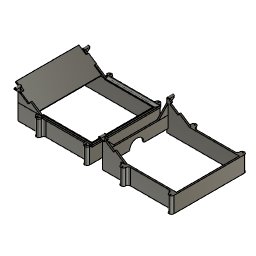
Led backlight edge holder (Autodesk Fusion 360 design; units mm, degrees)
Autodesk Fusion 360 part; units mm, degrees
note: some values were not read from the file. Chosen so that the rebuilt part matches the saved one: which pieces of a blend or face edit are solid. Set by a fixed rule: which sketch regions a step uses.
sketch "Sketch1" plane through (0, 0, 0) normal (0, 0, 1) x (1, 0, 0) in component "Base"
  line L0 (110, 0) -> (110, 126)
  line L1 (110, 126) -> (0, 126)
  line L2 (0, 126) -> (0, 0)
  line L3 (112, 128) -> (-35, 128)
  line L4 (-35, 128) -> (-35, -2)
  line L5 (-35, -2) -> (112, -2)
  line L6 (112, -2) -> (112, 128)
  line L7 (-45, 126) -> (-45, 0)
  line L8 (0, 0) -> (0, 126)
  line L9 (115, 131) -> (-38, 131)
  line L10 (-38, 131) -> (-38, -5)
  line L11 (-38, -5) -> (115, -5)
  line L12 (115, -5) -> (115, 131)
  line L13 (-35, -2) -> (-38, -2)
  line L14 (-35, 128) -> (-38, 128)
  line L15 (-38, 0) -> (-45, 0)
  line L16 (-45, 0) -> (-45, 126)
  line L17 (-45, 126) -> (-38, 126)
  line L18 (110, 0) -> (0, 0)
  line L19 (115, -5) -> (105, -5)
  line L20 (105, -5) -> (105, -15)
  line L21 (105, -15) -> (115, -15)
  line L22 (115, -15) -> (115, -5)
  line L23 (115, 131) -> (105, 131)
  line L24 (105, 131) -> (105, 141)
  line L25 (105, 141) -> (115, 141)
  line L26 (115, 141) -> (115, 131)
  line L27 (15, -5) -> (5, -5)
  line L28 (5, -5) -> (5, -15)
  line L29 (5, -15) -> (15, -15)
  line L30 (15, -15) -> (15, -5)
  line L31 (5, 131) -> (5, 141)
  line L32 (5, 141) -> (15, 141)
  line L33 (15, 141) -> (15, 131)
  line L34 (15, 131) -> (5, 131)
  circle A0 centre (10, -12) radius 1
  circle A1 centre (110, -12) radius 1
  circle A2 centre (110, 138) radius 1
  circle A3 centre (10, 138) radius 1
  dimension "d4" = 110
  dimension "d5" = 126
  dimension "d8" = 147
  dimension "d9" = 130
  dimension "d11" = 153
  dimension "d12" = 136
  constraint vertical L0
  constraint horizontal L1
  constraint vertical L2
  constraint coincident L2.end L8.start
  constraint horizontal L3
  constraint vertical L4
  constraint horizontal L5
  constraint vertical L6
  constraint vertical L7
  constraint vertical L8
  constraint horizontal L9
  constraint vertical L10
  constraint horizontal L11
  constraint vertical L12
  constraint coincident L10 L13.end
  constraint perpendicular L10 L13
  constraint coincident L10 L14.end
  constraint perpendicular L10 L14
  constraint coincident L10 L15.start
  constraint coincident L10 L17.end
  constraint perpendicular L2 L18
  constraint horizontal L19
  constraint vertical L20
  constraint horizontal L21
  constraint vertical L22
  constraint horizontal L23
  constraint vertical L24
  constraint horizontal L25
  constraint vertical L26
  constraint horizontal L27
  constraint vertical L28
  constraint horizontal L29
  constraint vertical L30
  constraint horizontal L34
  constraint vertical L31
  constraint horizontal L32
  constraint vertical L33
  measures "d4" distance of L2.end L0.start
  measures "d5" distance of L2.end L1.end
  measures "d8" distance of L3.start L3.end
  measures "d9" distance of L3.start L5.end
  measures "d11" distance of L9.start L9.end
  measures "d12" distance of L9.start L11.end
extrude "Extrude1" add sketch "Sketch1" along normal blind 30 contours L3 L5 L6 L9 L10 L11 L12 L13 L14 L19 L23 L27 L34 makes body 1 in component "Base"
extrude "Extrude2" add sketch "Sketch1" along normal blind 30 contours L4 L10 L13 L14 bodies 1 in component "Base"
extrude "Extrude3" cut sketch "Sketch1" along normal blind 6 contours L4 L10 L13 L14 bodies 1 in component "Base"
sketch "Sketch2" plane through (0, 131, 0) normal (0, 1, 0) x (-1, 0, 0) in component "Ramp holder"
  line L0 (-115, 0) -> (38, 0)
  line L1 (38, 0) -> (38, 30)
  line L2 (38, 30) -> (-115, 30)
  line L3 (-115, 30) -> (-115, 0)
  line L4 (14.7979, 39.9099) -> (31.5016, 50.9092)
  line L5 (14.7979, 39.9099) -> (12.048, 44.0859)
  line L6 (31.5016, 50.9092) -> (28.7518, 55.0852)
  circle A0 centre (35.72, 59.5131) radius 0.9615
  circle A1 centre (35.72, 59.5131) radius 1.3
  circle A2 centre (35.72, 59.5131) radius 2.3
  line L7 (38.02, 57.0131) -> (38.0199, 59.4994)
  line L8 (33.42, 57.0131) -> (33.42, 59.5131)
  line L9 (33.42, 57.0131) -> (38.02, 57.0131)
  line L10 (38, 30, 0) -> (38, 30, -136)
  line L11 (38, 30, 0) -> (38, 30, -23)
  line L12 (38, 30) -> (-9.3431, 30)
  line L13 (-9.3431, 30) -> (12.048, 44.0859)
  line L14 (38, 30) -> (38.0199, 30.0131)
  line L15 (38, 30) -> (38.02, 57.0131)
  line L16 (28.7518, 55.0852) -> (33.42, 58.1591)
  line L17 (38.0155, 50.9044, 0) -> (38.0155, 50.9044, -3)
  line L18 (38.0155, 50.9044, -3) -> (38, 30, -23)
  line L19 (38, 30) -> (38.0155, 50.9044)
  dimension "d28" = 5
  dimension "d67" = 23
  dimension "d98" = 3
  constraint concentric A0 A1
  constraint concentric A1 A2
  constraint coincident A2 L7.end
  constraint coincident A2 L8.end
  constraint tangent A2 L8
  constraint horizontal L9
  constraint coincident L1.end L2.start
  constraint coincident L2 L12.end
  constraint perpendicular L5 L13
  constraint coincident L8 L16.end
  constraint coincident L15 L19.end
  measures "d28" distance of L4.end L6.end
  measures "d67" distance of L1.end L2.start
extrude "Extrude5" add sketch "Sketch2" against normal blind 3 separate body contours L2 L4 L5 L6 L8 L9 L12 L13 L15 L16 L19 | A2 L7 L8 L9 | A2 | A1 makes body 2 in component "Base"
extrude "Extrude6" cut sketch "Sketch2" against normal blind 2 contours A1 bodies 2 in component "Base"
extrude "Extrude7" add sketch "Sketch2" along normal blind 8 contours A2 L7 L8 L9 | A2 bodies 2 in component "Base"
fillet "Fillet3" radius 8 tangency weight 0.3 1 edges at (-35.72, 131, 57.0131) on bodies 2 in component "Base"
fillet "Fillet2" radius 1.25 tangency weight 0.8 1 edges at (-35.72, 139, 57.0131) on bodies 2 in component "Base"
sketch "Sketch2 (curves on the plane with normal -1, 0, -0.0007 at 37.9778 mm)" plane through (-37.9778, 131, -0.0281) normal (-1, 0, -0.00074) x (-0.00074, 0, 1)
  line L0 (30.0281, 0) -> (30.0281, -136)
  line L1 (30.0281, 0) -> (30.0281, -23)
  line L2 (30.0281, 0) -> (57.0412, 0)
  line L3 (50.9325, 0) -> (50.9325, -3)
  line L4 (50.9325, -3) -> (30.0281, -23)
  line L5 (30.0281, 0) -> (50.9325, 0)
extrude "Extrude9" add sketch "Sketch2 (curves on the plane with normal -1, 0, -0.0007 at 37.9778 mm)" against normal blind 3 bodies 2 in component "Base"
sketch "Sketch1 (2)" plane through (0, 0, 0) normal (0, 0, 1) x (1, 0, 0) in component "Ramp"
  line L0 (-78, 135) -> (-78, 140)
  line L1 (-78, 140) -> (-98, 140)
  line L2 (-98, 140) -> (-98, 135)
  line L3 (-98, 5) -> (-98, 0)
  line L4 (-98, 0) -> (-78, 0)
  line L5 (-78, 0) -> (-78, 5)
  line L6 (-98, 135) -> (-116, 135)
  line L7 (-98, 5) -> (-116, 5)
  line L8 (-116, 135) -> (-116, 5)
  line L9 (-78, 5) -> (-60, 5)
  line L10 (-60, 5) -> (-60, 135)
  line L11 (-60, 135) -> (-78, 135)
  dimension "d72" = 5
  dimension "d73" = 20
  dimension "d101" = 18
  dimension "d102" = 18
  dimension "d103" = 18
  constraint perpendicular L0 L1
  constraint perpendicular L1 L2
  constraint perpendicular L3 L4
  constraint perpendicular L4 L5
  constraint perpendicular L2 L6
  constraint perpendicular L3 L7
  constraint perpendicular L7 L8
  constraint perpendicular L5 L9
  constraint perpendicular L9 L10
  constraint perpendicular L0 L11
  measures "d72" distance of L0.start L0.end
  measures "d73" distance of L0.end L1.end
  measures "d101" distance of L2.end L6.end
  measures "d102" distance of L3.start L7.end
  measures "d103" distance of L5.end L9.end
extrude "Extrude1'" add sketch "Sketch1 (2)" along normal blind 3 separate body makes body 3 in component "Ramp"
copy_body "CutPasteBodies1" bodies 2 removing the originals makes body 4 in component "Ramp holder"
mirror "MirrorComponent4" about plane through (0, 0, 0) normal (0, 0, 1) of bodies 4 makes body 5 in component "Ramp holder(Mirror)"
extrude "Extrude1''" add sketch "Sketch1" along normal blind 30 contours L9 L31 L32 L33 L34 | L11 L27 L28 L29 L30 | L9 L23 L24 L25 L26 | L11 L19 L20 L21 L22 bodies 1 in component "Base"
fillet "Fillet1" radius 5 14 edges at (105, 141, 15) (105, 131, 15) (115, 141, 15) (15, 131, 15) (15, 141, 15) (5, 131, 15) (5, 141, 15) (15, -5, 15) (15, -15, 15) (5, -15, 15) (5, -5, 15) (105, -5, 15) (105, -15, 15) (115, -15, 15) on bodies 1 in component "Base"
sketch "Sketch1 (3)" plane through (0, 0, 0) normal (0, 0, 1) x (1, 0, 0) in component "Edge"
  line L0 (105, 141) -> (115, 141)
  line L1 (5, 141) -> (15, 141)
  line L2 (5, -15) -> (15, -15)
  line L3 (105, -15) -> (115, -15)
  circle A0 centre (110, -12) radius 1.25
  circle A1 centre (10, -12) radius 1.25
  circle A2 centre (10, 138) radius 1.25
  circle A3 centre (110, 138) radius 1.25
  line L4 (10, -8) -> (118, -8)
  line L5 (118, -8) -> (118, 134)
  line L6 (118, 134) -> (10, 134)
  line L7 (10, -8) -> (10, -8.5)
  line L8 (10, -8.5) -> (118.5, -8.5)
  line L9 (118.5, -8.5) -> (118.5, 134.5)
  line L10 (118.5, 134.5) -> (10, 134.5)
  line L11 (115, -15) -> (115, -8.5)
  line L12 (105, -15) -> (105, -8.5)
  line L13 (15, -15) -> (15, -8.5)
  line L14 (5, -15) -> (5, -8.5)
  line L15 (5, -8.5) -> (10, -8.5)
  line L16 (105, 141) -> (105, 134.5)
  line L17 (115, 141) -> (115, 134.5)
  line L18 (10, 134) -> (10, 134.5)
  line L19 (15, 141) -> (15, 134.5)
  line L20 (5, 141) -> (5, 134.5)
  line L21 (5, 134.5) -> (10, 134.5)
  line L22 (10, 0) -> (110, 0)
  line L23 (110, 0) -> (110, 126)
  line L24 (110, 126) -> (10, 126)
  line L25 (10, -8) -> (10, 0)
  line L26 (10, 126) -> (10, 134)
  dimension "d116" = 2.5
  dimension "d117" = 2.5
  dimension "d118" = 2.5
  dimension "d119" = 2.5
  dimension "d132" = 108
  dimension "d133" = 142
  dimension "d134" = 108.5
  dimension "d135" = 143
  constraint horizontal L0
  constraint horizontal L1
  constraint horizontal L2
  constraint horizontal L3
  constraint horizontal L4
  constraint vertical L5
  constraint horizontal L6
  constraint perpendicular L4 L7
  constraint horizontal L8
  constraint vertical L9
  constraint horizontal L10
  constraint coincident L8 L11.end
  constraint perpendicular L8 L11
  constraint coincident L8 L12.end
  constraint perpendicular L8 L12
  constraint coincident L8 L13.end
  constraint perpendicular L8 L13
  constraint perpendicular L2 L14
  constraint coincident L10 L16.end
  constraint perpendicular L10 L16
  constraint coincident L10 L17.end
  constraint perpendicular L10 L17
  constraint perpendicular L10 L18
  constraint coincident L10 L19.end
  constraint perpendicular L10 L19
  constraint perpendicular L1 L20
  constraint perpendicular L18 L21
  constraint perpendicular L22 L25
  constraint perpendicular L24 L26
  measures "d116" diameter of A0
  measures "d117" diameter of A1
  measures "d118" diameter of A2
  measures "d119" diameter of A3
  measures "d132" distance of L4.start L4.end
  measures "d133" distance of L4.start L6.end
  measures "d134" distance of L7.end L8.end
  measures "d135" distance of L7.end L10.end
extrude "Extrude4" add sketch "Sketch1 (3)" along normal blind 3 separate body contours L0 L10 L16 L17 | L4 L5 L6 L7 L8 L9 L10 L18 | L1 L10 L19 L20 L21 | L3 L8 L11 L12 | L2 L8 L13 L14 L15 makes body 6 in component "Edge"
extrude "Extrude6'" add sketch "Sketch1 (3)" along normal blind 0.2 contours L4 L5 L6 L22 L23 L24 L25 L26 bodies 6 in component "Edge"
fillet "Fillet8" radius 1 3 edges at (60, 126, 0.2) (110, 63, 0.2) (60, 0, 0.2) on bodies 6 in component "Edge"
fillet "Fillet9" radius 11.15 3 edges at (64, -8, 0.2) (118, 63, 0.2) (64, 134, 0.2) on bodies 6 in component "Edge"
fillet "Fillet11" radius 5 8 edges at (115, -15, 1.5) (105, -15, 1.5) (15, -15, 1.5) (5, -15, 1.5) (115, 141, 1.5) (105, 141, 1.5) (15, 141, 1.5) (5, 141, 1.5) on bodies 6 in component "Edge"
fillet "Fillet12" radius 1.5 8 edges at (5, 134.5, 1.5) (15, 134.5, 1.5) (105, 134.5, 1.5) (115, 134.5, 1.5) (115, -8.5, 1.5) (105, -8.5, 1.5) (5, -8.5, 1.5) (15, -8.5, 1.5) on bodies 6 in component "Edge"
fillet "Fillet13" radius 3.5 2 edges at (10, -8.5, 1.5) (10, 134.5, 1.5) on bodies 6 in component "Edge"
fillet "Fillet14" radius 0.5 2 edges at (118.5, 134.5, 1.5) (118.5, -8.5, 1.5) on bodies 6 in component "Edge"
move_face "OffsetFaces1" offset 3 1 faces at (108.8146, -6.9759, 0) on bodies 1 in component "Base"
sketch "Sketch1 (1)" plane through (-38, 0, 0) normal (-1, 0, 0) x (0, -1, 0) in component "Base"
  line L0 (2, 6) -> (2, -3)
  line L1 (2, -3) -> (5, -3)
  line L2 (5, -3) -> (5, 30)
  line L3 (5, 30) -> (-131, 30)
  line L4 (-131, 30) -> (-131, -3)
  line L5 (-131, -3) -> (-128, -3)
  line L6 (-128, -3) -> (-128, 6)
  line L7 (-128, 6) -> (2, 6)
  arc A0 (-48, 6) -> (-78, 6) centre (-63, 6) ccw
  dimension "d175" = 15
  constraint midpoint L7 A0.centre
  measures "d175" radius of A0
extrude "Extrude3'" cut sketch "Sketch1 (1)" against normal blind 3 contours L7 A0 bodies 1 in component "Base"
combine "Combine1" operation add target body 1 tool bodies 4 5 body 5 seen with x (1, 0, 0) y (0, -1, 0) z (0, 0, -1) at (0, 126, 0) keep tools result as body 7 in component "Led Backlight"
component "Base" placed x (1, 0, 0) y (0, 1, 0) z (0, 0, 1) at (0, 0, 0)
component "Ramp holder" placed x (1, 0, 0) y (0, 1, 0) z (0, 0, 1) at (0, 0, 0)
component "Ramp holder(Mirror)" placed x (1, 0, 0) y (0, -1, 0) z (0, 0, -1) at (0, 126, 0)
component "Ramp" placed x (1, 0, 0) y (0, 1, 0) z (0, 0, 1) at (0, 0, 0)
component "Ramp" placed x (0.835807, 0, -0.549023) y (0, 1, 0) z (0.549023, 0, 0.835807) at (50.4958, -7.1, -2.7605)
component "Edge" placed x (1, 0, 0) y (0, 1, 0) z (0, 0, 1) at (0, 0, 30)
component "Backlight edges" placed x (1, 0, 0) y (0, 1, 0) z (0, 0, 1) at (0, 0, 0)
component "Led Backlight" placed x (1, 0, 0) y (0, 1, 0) z (0, 0, 1) at (0, 0, 0)
